Autodesk Inventor part; units mm, degrees
(part 2 of 2)
sketch "Sketch26" plane through (0, 4, 0) normal (0, 1, 0) x (1, 0, 0)
  line L0 (-144.4, 168.6052) -> (-150.4, 168.6052) construction
  line L1 (-150.4, 168.6052) -> (-150.4, 105.7402) construction
  line L2 (-150.4, 105.7402) -> (-144.4, 105.7402) construction
  line L3 (-144.4, 105.7402) -> (-144.4, 100.6602) construction
  line L4 (-144.4, 100.6602) -> (-150.4, 100.6602) construction
  line L5 (-150.4, 100.6602) -> (-150.4, 37.7952) construction
  line L6 (-150.4, 37.7952) -> (-144.4, 37.7952) construction
  line L7 (-144.4, 37.7952) -> (-144.4, 32.7152) construction
  line L8 (-144.4, 32.7152) -> (-150.4, 32.7152) construction
  line L9 (-150.4, 32.7152) -> (-150.4, 2) construction
  line L10 (-150.4, 2) -> (-116.102, 2) construction
  line L11 (-116.102, 2) -> (-116.102, 8) construction
  line L12 (-116.102, 8) -> (-109.498, 8) construction
  line L13 (-109.498, 8) -> (-109.498, 2) construction
  line L14 (-109.498, 2) -> (-78.502, 2) construction
  line L15 (-78.502, 2) -> (-78.502, 8) construction
  line L16 (-78.502, 8) -> (-71.898, 8) construction
  line L17 (-71.898, 8) -> (-71.898, 2) construction
  line L18 (-71.898, 2) -> (-40.902, 2) construction
  line L19 (-40.902, 2) -> (-40.902, 8) construction
  line L20 (-40.902, 8) -> (-34.298, 8) construction
  line L21 (-34.298, 8) -> (-34.298, 2) construction
  line L22 (-34.298, 2) -> (-2, 2) construction
  line L23 (-2, 2) -> (-2, 226.6) construction
  line L24 (-2, 226.6) -> (-34.298, 226.6) construction
  line L25 (-34.298, 226.6) -> (-34.298, 220.6) construction
  line L26 (-34.298, 220.6) -> (-40.902, 220.6) construction
  line L27 (-40.902, 220.6) -> (-40.902, 226.6) construction
  line L28 (-40.902, 226.6) -> (-71.898, 226.6) construction
  line L29 (-71.898, 226.6) -> (-71.898, 220.6) construction
  line L30 (-71.898, 220.6) -> (-78.502, 220.6) construction
  line L31 (-78.502, 220.6) -> (-78.502, 226.6) construction
  line L32 (-78.502, 226.6) -> (-109.498, 226.6) construction
  line L33 (-109.498, 226.6) -> (-109.498, 220.6) construction
  line L34 (-109.498, 220.6) -> (-116.102, 220.6) construction
  line L35 (-116.102, 220.6) -> (-116.102, 226.6) construction
  line L36 (-116.102, 226.6) -> (-150.4, 226.6) construction
  line L37 (-150.4, 226.6) -> (-150.4, 173.6852) construction
  line L38 (-150.4, 173.6852) -> (-144.4, 173.6852) construction
  line L39 (-144.4, 173.6852) -> (-144.4, 168.6052) construction
  circle A0 centre (-87.934, 154.5) radius 3.25 construction
  circle A1 centre (-110.934, 212.5) radius 3.25 construction
  line L40 (-45, 152.425) -> (-45, 142.425) construction
  line L41 (-45, 142.425) -> (-55, 142.425) construction
  line L42 (-55, 142.425) -> (-55, 152.425) construction
  line L43 (-55, 152.425) -> (-45, 152.425) construction
  line L44 (-24.68, 142.425) -> (-34.68, 142.425) construction
  line L45 (-34.68, 142.425) -> (-34.68, 152.425) construction
  line L46 (-34.68, 152.425) -> (-24.68, 152.425) construction
  line L47 (-24.68, 152.425) -> (-24.68, 142.425) construction
  line L48 (-59.92, 197.85) -> (-61.92, 197.85) construction
  line L49 (-59.92, 197.85) -> (-59.92, 179.1) construction
  line L50 (-59.92, 179.1) -> (-4, 179.1) construction
  line L51 (-4, 179.1) -> (-4, 177.1) construction
  line L52 (-4, 177.1) -> (-61.92, 177.1) construction
  line L53 (-61.92, 177.1) -> (-61.92, 197.85) construction
  line L54 (-120.934, 157.75) -> (-110.934, 157.75) construction
  arc A2 (-110.934, 151.25) -> (-110.934, 157.75) centre (-110.934, 154.5) ccw construction
  line L55 (-110.934, 151.25) -> (-120.934, 151.25) construction
  line L56 (-120.934, 151.25) -> (-120.934, 157.75) construction
  line L57 (-77.934, 209.25) -> (-87.934, 209.25) construction
  arc A3 (-87.934, 215.75) -> (-87.934, 209.25) centre (-87.934, 212.5) ccw construction
  line L58 (-87.934, 215.75) -> (-77.934, 215.75) construction
  line L59 (-77.934, 215.75) -> (-77.934, 209.25) construction
  line L60 (-61.684, 114) -> (-55, 114) construction
  line L61 (-55, 114) -> (-55, 121.75) construction
  line L62 (-55, 121.75) -> (-13.4, 121.75) construction
  line L63 (-13.4, 121.75) -> (-13.4, 127.75) construction
  line L64 (-13.4, 127.75) -> (-7.4, 127.75) construction
  line L65 (-7.4, 127.75) -> (-7.4, 118.35) construction
  line L66 (-7.4, 118.35) -> (-9, 118.35) construction
  line L67 (-9, 118.35) -> (-9, 12.5) construction
  line L68 (-9, 12.5) -> (-50.6, 12.5) construction
  line L69 (-50.6, 12.5) -> (-50.6, 6.5) construction
  line L70 (-50.6, 6.5) -> (-56.6, 6.5) construction
  line L71 (-56.6, 6.5) -> (-56.6, 15.9) construction
  line L72 (-56.6, 15.9) -> (-55, 15.9) construction
  line L73 (-55, 15.9) -> (-55, 40) construction
  line L74 (-55, 40) -> (-61.684, 40) construction
  line L75 (-61.684, 40) -> (-61.684, 15.5) construction
  arc A4 (-65.934, 11.25) -> (-61.684, 15.5) centre (-62.934, 12.5) ccw construction
  line L76 (-65.934, 11.25) -> (-107.934, 11.25) construction
  arc A5 (-112.184, 15.5) -> (-107.934, 11.25) centre (-110.934, 12.5) ccw construction
  line L77 (-112.184, 15.5) -> (-112.184, 138.5) construction
  arc A6 (-107.934, 142.75) -> (-112.184, 138.5) centre (-110.934, 141.5) ccw construction
  line L78 (-107.934, 142.75) -> (-65.934, 142.75) construction
  arc A7 (-61.684, 138.5) -> (-65.934, 142.75) centre (-62.934, 141.5) ccw construction
  line L79 (-64.184, 138.5) -> (-61.684, 138.5) construction
  arc A8 (-65.934, 140.25) -> (-64.184, 138.5) centre (-62.934, 141.5) ccw construction
  line L80 (-65.934, 140.25) -> (-107.934, 140.25) construction
  arc A9 (-109.684, 138.5) -> (-107.934, 140.25) centre (-110.934, 141.5) ccw construction
  line L81 (-109.684, 138.5) -> (-109.684, 15.5) construction
  arc A10 (-107.934, 13.75) -> (-109.684, 15.5) centre (-110.934, 12.5) ccw construction
  line L82 (-107.934, 13.75) -> (-65.934, 13.75) construction
  arc A11 (-64.184, 15.5) -> (-65.934, 13.75) centre (-62.934, 12.5) ccw construction
  line L83 (-64.184, 15.5) -> (-64.184, 57) construction
  line L84 (-61.684, 57) -> (-64.184, 57) construction
  line L85 (-61.684, 57) -> (-61.684, 47) construction
  line L86 (-61.684, 47) -> (-55, 47) construction
  line L87 (-55, 47) -> (-55, 107) construction
  line L88 (-55, 107) -> (-61.684, 107) construction
  line L89 (-61.684, 107) -> (-61.684, 97) construction
  line L90 (-64.184, 97) -> (-61.684, 97) construction
  line L91 (-64.184, 97) -> (-64.184, 125.5) construction
  line L92 (-61.684, 125.5) -> (-64.184, 125.5) construction
  line L93 (-61.684, 125.5) -> (-61.684, 114) construction
  line L94 (-61.92, 205.85) -> (-61.92, 224.6) construction
  line L95 (-61.92, 224.6) -> (-59.92, 224.6) construction
  line L96 (-59.92, 224.6) -> (-59.92, 205.85) construction
  line L97 (-61.92, 205.85) -> (-59.92, 205.85) construction
  line L98 (-144.4, 8) -> (-2, 8) construction
  line L99 (-2, 8) -> (-2, 220.6) construction
  line L100 (-2, 220.6) -> (-144.4, 220.6) construction
  line L101 (-144.4, 220.6) -> (-144.4, 8) construction
  line L102 (-140.4, 12) -> (-6, 12) construction
  line L103 (-6, 12) -> (-6, 216.6) construction
  line L104 (-6, 216.6) -> (-140.4, 216.6) construction
  line L105 (-140.4, 216.6) -> (-140.4, 12) construction
  line L106 (-140.4, 12) -> (-2, 12)
  line L107 (-2, 12) -> (-2, 216.6)
  line L108 (-2, 216.6) -> (-140.4, 216.6)
  line L109 (-140.4, 216.6) -> (-140.4, 12)
  point P0 (0, 0)
  dimension "d181" = 4
  constraints: 24 end point, 6 parallel, 3 perpendicular, 3 point on line, 2 horizontal, 3 other
  measures "d181" distance between parallel lines of L101 L105
extrude "Extrusion25" cut sketch "Sketch26" along normal mid plane 44.925
sketch "Sketch27" plane through (0, 16, 0) normal (0, 1, 0) x (1, 0, 0)
  line L0 (-155.6026, 232.387) -> (5.657, 232.387)
  line L1 (5.657, 232.387) -> (5.657, -6.1958)
  line L2 (5.657, -6.1958) -> (-155.6026, -6.1958)
  line L3 (-155.6026, -6.1958) -> (-155.6026, 232.387)
  point P0 (0, 0)
  constraints: 8 end point, 2 parallel, 1 horizontal, 1 perpendicular
extrude "Extrusion26" cut sketch "Sketch27" against normal up to surface (12 mm away)
sketch "Sketch28" plane through (0, 4, 0) normal (0, 1, 0) x (1, 0, 0)
  line L0 (-140.4, 216.6) -> (-2, 216.6) construction
  line L1 (-2, 216.6) -> (-2, 226.6) construction
  line L2 (-2, 226.6) -> (-34.298, 226.6) construction
  line L3 (-34.298, 226.6) -> (-34.298, 220.6) construction
  line L4 (-34.298, 220.6) -> (-40.902, 220.6) construction
  line L5 (-40.902, 220.6) -> (-40.902, 226.6) construction
  line L6 (-40.902, 226.6) -> (-71.898, 226.6) construction
  line L7 (-71.898, 226.6) -> (-71.898, 220.6) construction
  line L8 (-71.898, 220.6) -> (-78.502, 220.6) construction
  line L9 (-78.502, 220.6) -> (-78.502, 226.6) construction
  line L10 (-78.502, 226.6) -> (-109.498, 226.6) construction
  line L11 (-109.498, 226.6) -> (-109.498, 220.6) construction
  line L12 (-109.498, 220.6) -> (-116.102, 220.6) construction
  line L13 (-116.102, 220.6) -> (-116.102, 226.6) construction
  line L14 (-116.102, 226.6) -> (-150.4, 226.6) construction
  line L15 (-150.4, 226.6) -> (-150.4, 173.6852) construction
  line L16 (-150.4, 173.6852) -> (-144.4, 173.6852) construction
  line L17 (-144.4, 173.6852) -> (-144.4, 168.6052) construction
  line L18 (-144.4, 168.6052) -> (-150.4, 168.6052) construction
  line L19 (-150.4, 168.6052) -> (-150.4, 105.7402) construction
  line L20 (-150.4, 105.7402) -> (-144.4, 105.7402) construction
  line L21 (-144.4, 105.7402) -> (-144.4, 100.6602) construction
  line L22 (-144.4, 100.6602) -> (-150.4, 100.6602) construction
  line L23 (-150.4, 100.6602) -> (-150.4, 37.7952) construction
  line L24 (-150.4, 37.7952) -> (-144.4, 37.7952) construction
  line L25 (-144.4, 37.7952) -> (-144.4, 32.7152) construction
  line L26 (-144.4, 32.7152) -> (-150.4, 32.7152) construction
  line L27 (-150.4, 32.7152) -> (-150.4, 2) construction
  line L28 (-150.4, 2) -> (-116.102, 2) construction
  line L29 (-116.102, 2) -> (-116.102, 8) construction
  line L30 (-116.102, 8) -> (-109.498, 8) construction
  line L31 (-109.498, 8) -> (-109.498, 2) construction
  line L32 (-109.498, 2) -> (-78.502, 2) construction
  line L33 (-78.502, 2) -> (-78.502, 8) construction
  line L34 (-78.502, 8) -> (-71.898, 8) construction
  line L35 (-71.898, 8) -> (-71.898, 2) construction
  line L36 (-71.898, 2) -> (-40.902, 2) construction
  line L37 (-40.902, 2) -> (-40.902, 8) construction
  line L38 (-40.902, 8) -> (-34.298, 8) construction
  line L39 (-34.298, 8) -> (-34.298, 2) construction
  line L40 (-34.298, 2) -> (-2, 2) construction
  line L41 (-2, 2) -> (-2, 12) construction
  line L42 (-2, 12) -> (-140.4, 12) construction
  line L43 (-140.4, 12) -> (-140.4, 216.6) construction
  circle A0 centre (-53.6, 9.5) radius 2.25 construction
  line L44 (-2, 12) -> (11.0148, 12) construction
  line L45 (11.0148, 12) -> (11.0148, 216.6) construction
  line L46 (11.0148, 216.6) -> (-2, 216.6) construction
  line L47 (-2, 216.6) -> (-2, 12) construction
  line L48 (-2, 12) -> (11.0148, 12)
  line L49 (11.0148, 12) -> (11.0148, 216.6)
  line L50 (11.0148, 216.6) -> (-2, 216.6)
  line L51 (-2, 216.6) -> (-2, 12)
  point P0 (0, 0)
  constraints: 16 end point, 4 parallel, 2 horizontal, 2 perpendicular
extrude "Extrusion27" cut sketch "Sketch28" against normal blind 10
sketch "Sketch29" plane through (0, 4, 0) normal (0, 1, 0) x (1, 0, 0)
  circle A0 centre (-53.6, 9.5) radius 2.25 projected
  point P0 (0, 0)
extrude "Extrusion28" add sketch "Sketch29" against normal up to surface (0.5 mm away)
body "Solid1"
